Autodesk Inventor part; units mm, degrees
(part 2 of 2)
extrude "Extrusion61" cut sketch "Sketch85" against normal blind 15.5
sketch "Sketch86" plane through (0, 100, 0) normal (0, 1, 0) x (1, 0, 0)
  line L0 (-10, 136) -> (0, 136) projected
  line L1 (0, 136) -> (0, 10) projected
  line L2 (-10, 136) -> (0, 136)
  line L3 (0, 136) -> (0, 126)
  line L4 (0, 126) -> (-10, 126)
  line L5 (-10, 126) -> (-10, 136)
  line L6 (-4, 92) -> (-6, 92) projected
  line L7 (-6, 92) -> (-4, 92)
  line L8 (-4, 92) -> (-4, 128)
  line L9 (-4, 128) -> (-6, 128)
  line L10 (-6, 128) -> (-6, 92)
  line L11 (-10, 90) -> (-6, 90) projected
  line L12 (0, 126) -> (-10, 126)
  line L13 (-10, 126) -> (-10, 90)
  line L14 (-10, 90) -> (0, 90)
  line L15 (0, 90) -> (0, 126)
  line L16 (-4, 128) -> (-3.8, 128)
  line L17 (-3.8, 128) -> (-3.8, 126)
  line L18 (-3.8, 126) -> (-4, 126)
  line L19 (-4, 126) -> (-4, 128)
  line L20 (-4, 18) -> (-6, 18) projected
  line L21 (0, 20) -> (-4, 20) projected
  line L22 (-4, 18) -> (-3.8, 18)
  line L23 (-3.8, 18) -> (-3.8, 20)
  line L24 (-3.8, 20) -> (-4, 20)
  line L25 (-4, 20) -> (-4, 18)
  point P0 (0, 0)
  point P1 (-6, 126)
  point P2 (0, 90)
  dimension "d253" = 10
  dimension "d254" = 36
  dimension "d255" = 0.2
  dimension "d256" = 0.2
  constraints: 40 end point, 10 parallel, 5 horizontal, 5 perpendicular, 3 point on line
  measures "d253" distance of L2.end L3.end
  measures "d254" distance of L8.end L7.end
  measures "d255" distance of L17.end L18.end
  measures "d256" distance of L24.end L23.end
extrude "Extrusion62" cut sketch "Sketch86" against normal up to surface (40 mm away) contours L23 L22 L25 L21 | L4 L10 L6 L8 L1 L14 L11 L13 | L10 L9 L8 L4 | L4 L8 L6 L10 | L4 L8 L16 L17
sketch "Sketch87" plane through (5.7402, 50, -86) normal (0, 0, -1) x (-1, 0, 0)
  line L0 (1.7402, 0) -> (1.7402, 1.4916) projected
  line L1 (1.7402, 0) -> (-1.0957, 0)
  line L2 (-1.0957, 0) -> (-1.0957, 2.9424)
  line L3 (-1.0957, 2.9424) -> (1.7402, 2.9424)
  line L4 (1.7402, 2.9424) -> (1.7402, 0)
  line L5 (1.7402, 1.4916) -> (0, 0)
  point P0 (5.7402, -50)
  constraints: 10 end point, 2 parallel, 1 horizontal, 1 perpendicular
extrude "Extrusion63" add sketch "Sketch87" along normal blind 27.5 contours L1 L5 L0
sketch "Sketch88" plane through (4, 57, -100) normal (0, 0, -1) x (-1, 0, 0)
  line L0 (-14.5, -12) -> (-14.5, 0) projected
  line L1 (-12.5, -7) -> (-12.5, 0) projected
  line L2 (-14.5, 0) -> (-12.5, 0)
  line L3 (-12.5, 0) -> (-12.5, -7)
  line L4 (-12.5, -7) -> (-14.5, -7)
  line L5 (-14.5, -7) -> (-14.5, 0)
  line L6 (0, -5.5084) -> (0, 0) projected
  line L7 (2, -7) -> (2, 0) projected
  line L8 (0, 0) -> (2, 0)
  line L9 (2, 0) -> (2, -7)
  line L10 (2, -7) -> (0, -7)
  line L11 (0, -7) -> (0, 0)
  line L12 (2, -7) -> (4, -7) projected
  line L13 (1.7402, -7) -> (0, -5.5084) projected
  line L14 (2, -7) -> (1.7402, -7)
  line L15 (1.7402, -7) -> (0, -5.5084)
  point P0 (4, -57)
  constraints: 20 end point, 4 parallel, 2 collinear, 2 horizontal, 2 perpendicular
extrude "Extrusion64" cut sketch "Sketch88" against normal blind 6.75 contours L0 L2 L1 L4 | L6 L8 L7 L10 L13
sketch "Sketch89" plane through (0, 57, 0) normal (0, 1, 0) x (1, 0, 0)
  point P0 (0, 0)
sketch "Sketch90" plane through (0, 50, 0) normal (0, 1, 0) x (1, 0, 0)
  line L0 (10, 94) -> (10, 47) projected
  line L1 (10, 94) -> (42.6887, 94)
  line L2 (42.6887, 94) -> (42.6887, 141.8669)
  line L3 (42.6887, 141.8669) -> (10, 141.8669)
  line L4 (10, 141.8669) -> (10, 94)
  line L5 (5.7402, 136) -> (18.5, 136) projected
  line L6 (10, 136) -> (12, 136)
  line L7 (12, 136) -> (12, 130)
  line L8 (12, 130) -> (10, 130)
  line L9 (10, 130) -> (10, 136)
  line L10 (12, 130) -> (24.5, 130)
  line L11 (24.5, 130) -> (24.5, 136)
  line L12 (24.5, 136) -> (12, 136)
  line L13 (12, 136) -> (12, 130)
  line L14 (24.5, 136) -> (26.5, 136)
  line L15 (26.5, 136) -> (26.5, 130)
  line L16 (26.5, 130) -> (24.5, 130)
  line L17 (24.5, 130) -> (24.5, 136)
  point P0 (0, 0)
  dimension "d263" = 12.5
  constraints: 32 end point, 8 parallel, 4 horizontal, 4 perpendicular, 2 point on line
  measures "d263" distance of L12.end L11.end
extrude "Extrusion65" add sketch "Sketch90" along normal up to surface (7 mm away) contours L4 L5 L7 L8 | L11 L14 L15 L16
sketch "Sketch91" plane through (18.5, 45, -94) normal (1, 0, 0) x (0, 0, -1)
  line L0 (42, 6.4916) -> (42, 5) projected
  line L1 (-164, 0) -> (42, 0) projected
  line L2 (42, 5) -> (36, 5)
  line L3 (36, 5) -> (36, 0)
  line L4 (36, 0) -> (42, 0)
  line L5 (42, 0) -> (42, 5)
  point P0 (-94, -45)
  point P1 (42, 0)
  dimension "d266" = 6
  constraints: 8 end point, 2 parallel, 1 horizontal, 1 perpendicular, 1 point on line
  measures "d266" distance of L4.end L3.end
extrude "Extrusion66" add sketch "Sketch91" along normal up to surface (8 mm away)
sketch "Sketch92" plane through (0, 50, 0) normal (0, 1, 0) x (1, 0, 0)
  line L0 (18.5, 130) -> (18.5, 94) projected
  line L1 (10, 94) -> (18.5, 94)
  line L2 (18.5, 94) -> (18.5, 130)
  line L3 (18.5, 130) -> (10, 130)
  line L4 (10, 130) -> (10, 94)
  point P0 (0, 0)
  constraints: 8 end point, 2 parallel, 1 horizontal, 1 perpendicular
extrude "Extrusion67" cut sketch "Sketch92" against normal blind 15.75
sketch "Sketch93" plane through (0, 50, 0) normal (0, 1, 0) x (1, 0, 0)
  point P0 (0, 0)
sketch "Sketch94" plane through (-10, 60, -20) normal (0, 1, 0) x (1, 0, 0)
  point P0 (10, -20)
sketch "Sketch95" plane through (0, 100, 0) normal (0, 1, 0) x (1, 0, 0)
  point P0 (0, 0)
sketch "Sketch96" plane through (12, 50, -130) normal (1, 0, 0) x (0, 0, -1)
  point P0 (-130, -50)
sketch "Sketch97" plane through (10, 45, -130) normal (0, 0, 1) x (1, 0, 0)
  point P0 (-10, -45)
sketch "Sketch98" plane through (0, 50, 0) normal (0, 1, 0) x (1, 0, 0)
  point P0 (0, 0)
equation "\"d1\" = d0"
equation "\"d2\" = 0.5 * d1"
equation "\"d3\" = 0.5 * d1"
equation "\"BendRadius\" = Thickness"
equation "\"BendReliefWidth\" = Thickness"
equation "\"BendReliefDepth\" = 0.5 * Thickness"
equation "\"CornerReliefSize\" = 4 * Thickness"
equation "\"MinimumRemnant\" = 2 * Thickness"
equation "\"TransitionRadius\" = BendRadius"
equation "\"JacobiRadiusSize\" = BendRadius"
equation "\"GapSize\" = Thickness"
equation "\"Thickness\" = 0.5"
body "Solid1"
